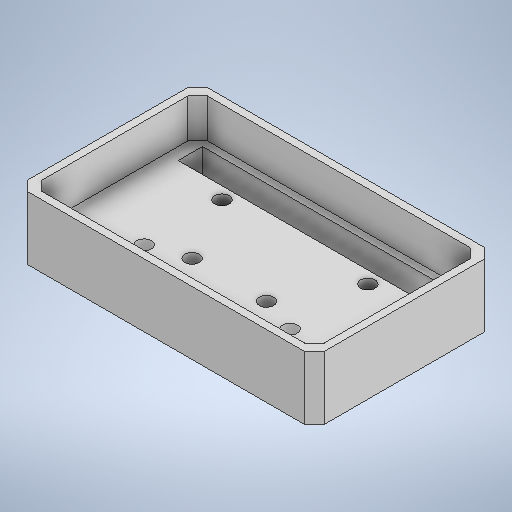
# Autodesk Inventor part: espTopLayer
Saved by Autodesk Inventor 2025 (Build 290162000, 162)
## iProperties
Created: 2025-04-09
Part Number: espTopLayer
Material: Genérico
Document SubType Name: Modeling
Designer: Ian
Density: 1 g/cm^3
Appearance: Padrão
Author: Ian
Autodesk Inventor part; units mm, degrees
ref_plane "YZ Plane" through (0, 0, 0) normal (1, 0, 0) x (0, 1, 0)
ref_plane "XZ Plane" through (0, 0, 0) normal (0, 1, 0) x (-1, 0, 0)
ref_plane "XY Plane" through (0, 0, 0) normal (0, 0, 1) x (1, 0, 0)
sketch "Esboço1" plane through (0, 0, 0) normal (0, 1, 0) x (-1, 0, 0)
  line L0 (-30.5, -18.5) -> (30.5, -18.5)
  line L1 (30.5, -18.5) -> (30.5, 18.5)
  line L2 (30.5, 18.5) -> (-30.5, 18.5)
  line L3 (-30.5, 18.5) -> (-30.5, -18.5)
  line L4 (-30.5, -18.5) -> (30.5, 18.5) construction
  line L5 (30.5, -18.5) -> (-30.5, 18.5) construction
  point P0 (0, 0)
  point P1 (0, 0)
  dimension "d2" = 61
  dimension "d3" = 37
  dimension "d6" = 0
  dimension "d7" = 0
  constraints: 12 end point, 2 midpoint, 2 parallel, 1 horizontal, 1 perpendicular, 1 other
  measures "d2" distance of L2.end L1.end
  measures "d3" distance of L1.end L0.end
  measures "d6" distance of point (0, 0) point (0, 0)
  measures "d7" distance of point (0, 0) point (0, 0)
extrude "Extrusão1" add sketch "Esboço1" along normal blind 5
sketch "Esboço3" plane through (0, 5, 0) normal (0, 1, 0) x (1, 0, 0)
  line L0 (29, -17) -> (-29, -17)
  line L1 (-29, -17) -> (-29, 17)
  line L2 (-29, 17) -> (29, 17)
  line L3 (29, 17) -> (29, -17)
  line L4 (29, -17) -> (-29, 17) construction
  line L5 (-29, -17) -> (29, 17) construction
  line L6 (-30.5, 18.5) -> (-30.5, -18.5) projected
  line L7 (30.5, -18.5) -> (-30.5, -18.5)
  line L8 (-30.5, -18.5) -> (-30.5, 18.5)
  line L9 (-30.5, 18.5) -> (30.5, 18.5)
  line L10 (30.5, 18.5) -> (30.5, -18.5)
  line L11 (30.5, -18.5) -> (-30.5, 18.5) construction
  line L12 (-30.5, -18.5) -> (30.5, 18.5) construction
  point P0 (0, 0)
  point P1 (-30.5, -18.5)
  dimension "d49" = 1.5
  dimension "d50" = 1.5
  constraints: 24 end point, 4 midpoint, 4 parallel, 2 horizontal, 2 perpendicular
  measures "d49" distance between parallel lines of L3 L10
  measures "d50" distance between parallel lines of L0 L7
extrude "Extrusão2" add sketch "Esboço3" along normal blind 8
chamfer "Chanfro1" distance 2 angle 45 4 edges at (-30.5, 6.5, -18.5) (-30.5, 6.5, 18.5) (30.5, 6.5, 18.5) (30.5, 6.5, -18.5)
chamfer "Chanfro2" distance 2 angle 45 4 edges at (29, 9, 17) (-29, 9, 17) (29, 9, -17) (-29, 9, -17)
sketch "Esboço4" plane through (0, 0, 0) normal (0, -1, 0) x (1, 0, 0)
  line L0 (26.5, 15.5) -> (-26.5, 15.5)
  line L1 (-26.5, 15.5) -> (-26.5, 10.5)
  line L2 (-26.5, 10.5) -> (26.5, 10.5)
  line L3 (26.5, 10.5) -> (26.5, 15.5)
  line L4 (-30.5, 18.5) -> (30.5, 18.5) projected
  line L5 (-30.5, -18.5) -> (-30.5, 18.5) projected
  line L6 (30.5, 18.5) -> (30.5, -18.5) projected
  line L7 (-26.5, -15.5) -> (26.5, -15.5)
  line L8 (26.5, -15.5) -> (26.5, -10.5)
  line L9 (26.5, -10.5) -> (-26.5, -10.5)
  line L10 (-26.5, -10.5) -> (-26.5, -15.5)
  line L11 (30.5, -18.5) -> (-30.5, -18.5) projected
  point P0 (0, 0)
  point P1 (-28.5, 18.5)
  point P2 (28.5, 18.5)
  point P3 (-30.5, -16.5)
  point P4 (-30.5, 16.5)
  point P5 (30.5, 16.5)
  point P6 (30.5, -16.5)
  point P7 (26.5, 13)
  point P8 (26.5, -13)
  point P9 (-26.5, -13)
  point P10 (28.5, -18.5)
  point P11 (-28.5, -18.5)
  dimension "d18" = 3
  dimension "d19" = 5
  dimension "d20" = 4
  dimension "d21" = 4
  dimension "d23" = 4
  dimension "d24" = 4
  dimension "d25" = 5
  dimension "d26" = 3
  constraints: 16 end point, 4 parallel, 3 midpoint, 2 horizontal, 2 perpendicular
  measures "d18" distance between parallel lines of L4 L0
  measures "d19" distance between parallel lines of L2 L0
  measures "d20" distance between parallel lines of L5 L1
  measures "d21" distance from line of L6 point (26.5, 13)
  measures "d23" distance from line of L6 point (26.5, -13)
  measures "d24" distance from line of L5 point (-26.5, -13)
  measures "d25" distance between parallel lines of L7 L9
  measures "d26" distance between parallel lines of L11 L7
extrude "Extrusão3" cut sketch "Esboço4" against normal through all contours L3 L2 L1 L0 | L10 L9 L8 L7
sketch "Esboço5" plane through (0, 0, 0) normal (0, -1, 0) x (1, 0, 0)
  line L0 (26.5, 10.5) -> (-26.5, 10.5) projected
  line L1 (-26.5, 10.5) -> (-26.5, 15.5) projected
  line L2 (-26.5, 15.5) -> (26.5, 15.5) projected
  line L3 (26.5, 15.5) -> (26.5, 10.5) projected
  line L4 (-26.5, -10.5) -> (26.5, -10.5) projected
  line L5 (26.5, -10.5) -> (26.5, -15.5) projected
  line L6 (26.5, -15.5) -> (-26.5, -15.5) projected
  line L7 (-26.5, -15.5) -> (-26.5, -10.5) projected
  line L8 (30.5, 16.5) -> (30.5, -16.5) projected
  line L9 (-28.5, 18.5) -> (28.5, 18.5) projected
  line L10 (-30.5, -16.5) -> (-30.5, 16.5) projected
  line L11 (28.5, -18.5) -> (-28.5, -18.5) projected
  circle A0 centre (15, 8) radius 1.5
  circle A1 centre (15, -8) radius 1.5
  circle A2 centre (-15, 8) radius 1.5
  circle A3 centre (-15, -8) radius 1.5
  line L12 (17.5, 10.5) -> (-17.5, 10.5)
  line L13 (-17.5, 10.5) -> (-17.5, -10.5)
  line L14 (-17.5, -10.5) -> (17.5, -10.5)
  line L15 (17.5, -10.5) -> (17.5, 10.5)
  line L16 (17.5, 10.5) -> (-17.5, -10.5) construction
  line L17 (-17.5, 10.5) -> (17.5, -10.5) construction
  line L18 (30.5, -16.5) -> (28.5, -18.5) projected
  line L19 (28.5, 18.5) -> (30.5, 16.5) projected
  line L20 (-30.5, 16.5) -> (-28.5, 18.5) projected
  line L21 (-28.5, -18.5) -> (-30.5, -16.5) projected
  circle A4 centre (-7.65, 5.5) radius 1.5
  circle A5 centre (7.65, 5.5) radius 1.5
  point P0 (0, 0)
  dimension "d31" = 3
  dimension "d35" = 2.5
  dimension "d36" = 2.5
  dimension "d38" = 2.5
  dimension "d42" = 35
  dimension "d43" = 2.5
  dimension "d44" = 2.5
  dimension "d45" = 21
  dimension "d46" = 2.5
  dimension "d47" = 2.5
  dimension "d48" = 2.5
  dimension "d51" = 3
  dimension "d52" = 3
  dimension "d55" = 5
  dimension "d56" = 5
  dimension "d58" = 15.3
  dimension "d59" = 9.85
  dimension "d60" = 9.85
  constraints: 12 end point, 6 centre point, 3 equal radius, 2 midpoint, 2 parallel, 1 horizontal, 1 perpendicular, 1 point on line
  measures "d31" diameter of A0
  measures "d35" distance from line of L4 A1.centre
  measures "d36" distance from line of L0 A2.centre
  measures "d38" distance from line of L4 A3.centre
  measures "d42" distance of L14.end L13.end
  measures "d43" distance from line of L12 A0.centre
  measures "d44" distance from line of L15 A0.centre
  measures "d45" distance of L12.end L13.end
  measures "d46" distance from line of L13 A2.centre
  measures "d47" distance from line of L13 A3.centre
  measures "d48" distance from line of L15 A1.centre
  measures "d51" diameter of A4
  measures "d52" diameter of A5
  measures "d55" distance from line of L12 A4.centre
  measures "d56" distance from line of L0 A5.centre
  measures "d58" distance of A4.centre A5.centre
  measures "d59" distance from line of L15 A5.centre
  measures "d60" distance from line of L13 A4.centre
extrude "Extrusão4" cut sketch "Esboço5" against normal through all contours A0 | A1 | A2 | A3 | A4 | A5
equation "\"d59\" = d60"
